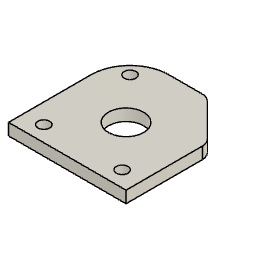
Magneto+Z+Spindel+Halter+oben+Teil2+RH+Deckel (Autodesk Fusion 360 design; units mm, degrees)
Autodesk Fusion 360 part; units mm, degrees
sketch "Skizze1" plane through (0, 0, 0) normal (0, 0, 1) x (1, 0, 0)
  line L0 (0, 0) -> (30, 0)
  line L1 (30, 0) -> (30, 30)
  line L2 (30, 30) -> (0, 30)
  line L3 (0, 30) -> (0, 0)
  line L4 (30, 20) -> (0, 20)
  line L5 (30, 10) -> (0, 10)
  dimension "d1" = 30
  dimension "d2" = 30
  constraint horizontal L0
  constraint vertical L1
  constraint horizontal L2
  constraint vertical L3
  constraint coincident L0.start L3.end
  measures "d1" distance of L0.start L0.end
  measures "d2" distance of L0.start L2.end
extrude "Extrusion1" add sketch "Skizze1" along normal blind 4 contours L0 L1 L3 L5 | L1 L2 L3 L4 makes body 1 at (10, 6.6667, 0) makes body 2 at (10, 26.6667, 0)
extrude "Extrusion2" add sketch "Skizze1" along normal blind 46 contours L1 L3 L4 L5 bodies 1 2
sketch "Skizze2" plane through (0, 10, 0) normal (0, -1, 0) x (1, 0, 0)
  line L0 (0, 4) -> (30, 4)
  line L1 (30, 4) -> (30, 46)
  line L2 (30, 46) -> (0, 46)
  line L3 (0, 46) -> (0, 4)
  circle A0 centre (15, 30) radius 11
  circle A1 centre (15, 30) radius 4.5
  line L4 (70, 14) -> (40, 14)
  line L5 (40, 14) -> (40, 46)
  line L6 (40, 46) -> (70, 46)
  line L7 (70, 46) -> (70, 14)
  circle A2 centre (55, 30) radius 4.5
  line L8 (40, 46) -> (45, 46)
  circle A3 centre (45, 41) radius 1.5
  circle A4 centre (65, 41) radius 1.5
  circle A5 centre (45, 19) radius 1.5
  circle A6 centre (65, 19) radius 1.5
  circle A7 centre (25, 41) radius 1.5
  circle A8 centre (5, 41) radius 1.5
  circle A9 centre (5, 19) radius 1.5
  circle A10 centre (25, 19) radius 1.5
  circle A11 centre (55, 30) radius 11
  point P0 (30, 0)
  dimension "d12" = 22
  dimension "d13" = 9
  dimension "d15" = 9
  dimension "d16" = 5
  dimension "d17" = 3
  dimension "d20" = 20
  dimension "d21" = -22
  dimension "d24" = 20
  dimension "d25" = -22
  dimension "d26" = 3
  dimension "d35" = 22
  constraint concentric A0 A1
  constraint horizontal L6
  constraint vertical L7
  constraint horizontal L4
  constraint vertical L5
  constraint coincident L6 L8.end
  constraint concentric A2 A11
  measures "d12" diameter of A0
  measures "d13" diameter of A1
  measures "d15" diameter of A2
  measures "d16" distance of L5.end L8.end
  measures "d17" diameter of A3
  measures "d26" diameter of A8
  measures "d35" diameter of A11
extrude "Extrusion3" cut sketch "Skizze2" against normal blind 55 contours A1 bodies 1
extrude "Extrusion4" cut sketch "Skizze2" against normal blind 54 contours A7 | A8 | A9 | A10 bodies 1
extrude "Extrusion5" cut sketch "Skizze2" against normal blind 7 contours A0 bodies 1
split "Teilen1" by plane through (0, 0, 4) normal (0, 0, 1) bodies 1 makes body 3 at (11.9784, 20, 8.6091)
move_body "Verschieben1" bodies 3 to x (1, 0, 0) y (0, 1, 0) z (0, 0, 1) at (0, 18, 0)
extrude "Extrusion8" add 1 faces at (10, 34.6667, 4) along direction (0, 0, -1) blind 4 on bodies 3 bodies 1 3
extrude "Extrusion9" cut 1 faces at (10, 0, 1.3333) along direction (0, 1, 0) blind 8 on bodies 1 bodies 1
sketch "Skizze3" plane through (0, 0, 4) normal (0, 0, 1) x (-1, 0, 0)
  line L0 (0, -8) -> (-30, -8)
  line L1 (-30, -8) -> (-30, -28)
  line L2 (-30, -28) -> (0, -28)
  line L3 (0, -28) -> (0, -8)
  circle A0 centre (-6, -18) radius 2.1
  circle A1 centre (-24, -18) radius 2.1
  dimension "d46" = 4.2
  dimension "d49" = 4.2
  measures "d46" diameter of A0
  measures "d49" diameter of A1
extrude "Extrusion10" cut sketch "Skizze3" against normal blind 10 contours A0 | A1 bodies 1
sketch "Skizze4" plane through (30, 0, 0) normal (1, 0, 0) x (0, 1, 0)
  line L0 (8, 4) -> (8, 0)
  line L1 (8, 0) -> (38, 0)
  line L2 (38, 0) -> (38, 46)
  line L3 (38, 46) -> (28, 46)
  line L4 (28, 46) -> (28, 4)
  line L5 (28, 4) -> (8, 4)
  line L6 (28, 4) -> (28, 14)
  line L7 (28, 4) -> (18, 4)
  line L8 (28, 14) -> (18, 4)
  line L9 (28, 4, -30) -> (28, 14, -30)
  line L10 (28, 14, -30) -> (28, 4, -30)
  line L11 (28, 4, -30) -> (18, 4, -30)
  line L12 (18, 4, -30) -> (28, 14, -30)
  point P0 (28, 4)
  point P1 (28, 4)
  point P2 (28, 4)
  dimension "d52" = 10
  dimension "d53" = 10
  dimension "d54" = 10
  constraint coincident P2 P1
  constraint coincident L4 L6.end
  constraint midpoint L5 L7.end
  measures "d52" distance of P2 L6.end
  measures "d53" distance of P2 L6.end
  measures "d54" distance of P2 L7.end
extrude "Extrusion11" add sketch "Skizze4" along normal blind 2 contours L9 L10 L11 L12 in plane through (0, 0, 0) normal (1, 0, 0) bodies 1
extrude "Extrusion12" add sketch "Skizze4" against normal blind 2 contours L4 L5 L6 L7 L8 bodies 1
fillet "Abrundung3" radius 3 1 edges at (30, 33, 46) on bodies 1
move_body "Verschieben2" bodies 1 to x (1, 0, 0) y (0, 0, -1) z (0, 1, 0) at (0, 38, 38)
sketch "Skizze5" plane through (0, 38, 0) normal (0, -1, 0) x (1, 0, 0)
  line L0 (0, 30) -> (0, 0)
  line L1 (0, 0) -> (30, 0)
  line L2 (30, 0) -> (30, 30)
  line L3 (30, 30) -> (0, 30)
  circle A0 centre (6, 20) radius 2.1
  circle A1 centre (24, 20) radius 2.1
  line L4 (15, 0) -> (21.5, 0)
  line L5 (21.5, 0) -> (8.5, 0)
  line L6 (8.5, 0) -> (21.5, 0)
  line L7 (21.5, 0) -> (21.5, 5)
  line L8 (21.5, 5) -> (8.5, 5)
  line L9 (8.5, 5) -> (8.5, 0)
  dimension "d64" = 13
  dimension "d65" = 13
  dimension "d66" = 5
  constraint midpoint L1 L4.start
  constraint parallel L4 L5
  constraint horizontal L6
  constraint vertical L7
  constraint horizontal L8
  constraint vertical L9
  measures "d64" distance of L4.end L5.end
  measures "d65" distance of L5.end L4.end
  measures "d66" distance of L5.end L8.end
extrude "Extrusion13" cut sketch "Skizze5" against normal blind 8 contours L1 L4 L5 L6 L7 L8 L9 bodies 1
sketch "Skizze6" plane through (0, 0, 10) normal (0, 0, 1) x (-1, 0, 0)
  line L0 (0, -84) -> (0, -52)
  line L1 (0, -52) -> (-2, -52)
  line L2 (-2, -52) -> (-2, -42)
  line L3 (-2, -42) -> (-28, -42)
  line L4 (-28, -42) -> (-28, -52)
  line L5 (-28, -52) -> (-30, -52)
  line L6 (-30, -52) -> (-30, -81)
  arc A0 (-30, -81) -> (-27, -84) centre (-27, -81) ccw
  line L7 (-27, -84) -> (0, -84)
  circle A1 centre (-15, -68) radius 11
  circle A2 centre (-5, -57) radius 1.5
  circle A3 centre (-25, -57) radius 1.5
  circle A4 centre (-5, -79) radius 1.5
  circle A5 centre (-25, -79) radius 1.5
  line L8 (-30, -73.7574) -> (-19.7574, -84)
  line L9 (-30, -73.7574) -> (-30, -84)
  line L10 (-30, -84) -> (-19.7574, -84)
  constraint coincident L6 L8.start
  constraint coincident L7 L8.end
  constraint parallel L6 L9
extrude "Extrusion14" cut sketch "Skizze6" against normal blind 24 contours L6 A0 L7 A5 L8 L9 L10 | A0 L9 L10 bodies 1
fillet "Abrundung4" radius 3 1 edges at (30, 73.7574, 5) on bodies 1
fillet "Abrundung5" radius 3 1 edges at (19.7574, 84, 5) on bodies 1
sketch "Skizze7" plane through (51.8787, 51.8787, 0) normal (0.707107, 0.707107, 0) x (-0.707107, 0.707107, 0)
  line L0 (44.1838, 0) -> (44.1838, 10)
  line L1 (44.1838, 10) -> (39.6739, 10)
  line L2 (39.6739, 10) -> (39.6739, 0)
  line L3 (39.6739, 0) -> (44.1838, 0)
  line L4 (44.1838, 0) -> (32.1838, 0)
  line L5 (32.1838, 0) -> (32.1838, 10)
  line L6 (32.1838, 10) -> (44.1838, 10)
  line L7 (44.1838, 10) -> (44.1838, 0)
  point P0 (32.1838, 10)
  constraint horizontal L4
  constraint vertical L5
  constraint horizontal L6
  constraint vertical L7
  constraint coincident P0 L5.end
  constraint coincident L0.start L3.end
extrude "Extrusion15" add sketch "Skizze7" against normal blind 2 bodies 1
extrude "Extrusion16" add 1 faces at (12.35, 42, 27.2729) along direction (0, 1, 0) blind 5 on bodies 1 bodies 1
extrude "Extrusion17" cut 1 faces at (17.1667, 38, 14.0478) along direction (0, 1, 0) blind 5 on bodies 1 bodies 1
extrude "Extrusion18" add 1 faces at (29.3333, 44.3333, 20) along direction (0, 0, -1) blind 6 on bodies 1 bodies 1
extrude "Extrusion19" add 1 faces at (1.3333, 44.3333, 20) along direction (0, 0, -1) blind 8 on bodies 1 bodies 1
sketch "Skizze8" plane through (0, 0, 3) normal (0, 0, 1) x (-1, 0, 0)
  circle A0 centre (-15, -68) radius 4.5
  circle A1 centre (-15, -68) radius 11
extrude "Extrusion20" cut 1 faces at (12.8333, 46, 1.6667) along direction (0, 1, 0) blind 5 on bodies 1 bodies 1
fillet "Abrundung6" radius 10 1 edges at (0, 84, 5) on bodies 1
fillet "Abrundung7" radius 3 2 edges at (0, 45, 30) (30, 45, 30) on bodies 1
extrude "Extrusion21" cut 1 faces at (11, 44.3333, 30) along direction (0, 0, -1) blind 56 on bodies 1 bodies 1
extrude "Extrusion22" cut 2 faces at (2, 43, 19) (28, 43, 19) along direction (0, 1, 0) blind 4 on bodies 1 bodies 1
extrude "Extrusion23" cut 1 faces at (3.5, 47, 5) along direction (0, 1, 0) blind 6 on bodies 1 bodies 1
extrude "Extrusion24" cut 1 faces at (12.8333, 51, 3.3333) along direction (0, 1, 0) blind 2 on bodies 1 bodies 1
extrude "Extrusion25" cut 1 faces at (28.5038, 63.4241, 10) along direction (0, 0, -1) blind 7 on bodies 1 bodies 1
